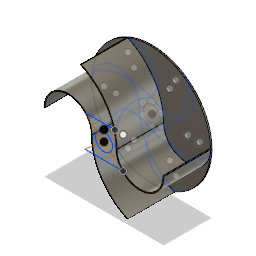
_Urinsky Turbine.044683ae-95bf-4561-8fff-8623c57a335d (Autodesk Fusion 360 design; units mm, degrees)
Autodesk Fusion 360 part; units mm, degrees
sketch "Sketch1" plane through (0, 0, 0) normal (0, 0, 1) x (1, 0, 0)
  circle A0 centre (0, 0) radius 125
  arc A1 (25, -0.0002) -> (-50.0002, 114.5643) centre (-100, -0.0002) ccw
  arc A2 (25, -0.0002) -> (125, -0.0004) centre (75, -0.0002) ccw
  arc A3 (-25, 0.0002) -> (50.0002, -114.5643) centre (100, 0.0002) ccw
  arc A4 (-25, 0.0002) -> (-125, 0.0004) centre (-75, 0.0002) ccw
  arc A5 (27, -0.0002) -> (-47.4802, 115.6314) centre (-100, -0.0002) ccw
  arc A6 (27, -0.0002) -> (123, -0.0004) centre (75, -0.0002) ccw
  arc A7 (-27, 0.0002) -> (47.4802, -115.6314) centre (100, 0.0002) ccw
  arc A8 (-27, 0.0002) -> (-123, 0.0004) centre (-75, 0.0002) ccw
  line L0 (50.0002, -114.5643) -> (47.4802, -115.6314)
  line L1 (-123, 0.0004) -> (-124.9746, -2.5191)
  line L2 (123, -0.0004) -> (124.9746, 2.5191)
  circle A9 centre (0, 0) radius 17.65
  circle A10 centre (0, 22) radius 1.5
  circle A11 centre (-19.0526, 11) radius 1.5
  circle A12 centre (-19.0526, -11) radius 1.5
  circle A13 centre (0, -22) radius 1.5
  circle A14 centre (19.0526, -11) radius 1.5
  circle A15 centre (19.0526, 11) radius 1.5
  line L3 (125, -0.0004) -> (124.9746, 2.5191)
  line L4 (-124.9746, -2.5191) -> (-125, 0.0004)
  line L5 (-50.0002, 114.5643) -> (-47.4802, 115.6314)
  arc A16 (-13.4998, 23.3828) -> (-61.4996, 106.5213) centre (-37.4998, 64.952) ccw
  line L6 (-62.4996, 108.2534) -> (-64.6689, 106.9717)
  line L7 (-61.4996, 106.5213) -> (-64.6689, 106.9717)
  line L8 (74.2155, 100.5836) -> (76.3997, 98.9348)
  line L9 (-74.2155, -100.5836) -> (-76.3997, -98.9348)
  arc A17 (12.4998, -21.6507) -> (62.4996, -108.2534) centre (37.4998, -64.952) ccw
  line L10 (64.6689, -106.9717) -> (62.4996, -108.2534)
  line L11 (61.4996, -106.5213) -> (64.6689, -106.9717)
  arc A18 (13.4998, -23.3828) -> (61.4996, -106.5213) centre (37.4998, -64.952) ccw
  arc A19 (-13.4998, 23.3828) -> (-76.3997, -98.9348) centre (50.0002, -86.6025) ccw
  arc A20 (-12.4998, 21.6507) -> (-74.2155, -100.5836) centre (50.0002, -86.6025) ccw
  arc A21 (-12.4998, 21.6507) -> (-62.4996, 108.2534) centre (-37.4998, 64.952) ccw
  arc A22 (12.4998, -21.6507) -> (74.2155, 100.5836) centre (-50.0002, 86.6025) ccw
  arc A23 (13.4998, -23.3828) -> (76.3997, 98.9348) centre (-50.0002, 86.6025) ccw
  arc A24 (-13.5002, -23.3826) -> (-61.5004, -106.5209) centre (-37.5002, -64.9518) ccw
  line L12 (-62.5004, -108.253) -> (-60.3057, -109.4907)
  line L13 (-61.5004, -106.5209) -> (-60.3057, -109.4907)
  line L14 (-124.2157, 13.9807) -> (-123.8799, 16.6967)
  line L15 (124.2157, -13.9807) -> (123.8799, -16.6967)
  arc A25 (12.5002, 21.6505) -> (62.5004, 108.253) centre (37.5002, 64.9518) ccw
  line L16 (60.3057, 109.4907) -> (62.5004, 108.253)
  line L17 (61.5004, 106.5209) -> (60.3057, 109.4907)
  arc A26 (13.5002, 23.3826) -> (61.5004, 106.5209) centre (37.5002, 64.9518) ccw
  arc A27 (-13.5002, -23.3826) -> (123.8799, -16.6967) centre (49.9998, 86.6026) ccw
  arc A28 (-12.5002, -21.6505) -> (124.2157, -13.9807) centre (49.9998, 86.6026) ccw
  arc A29 (-12.5002, -21.6505) -> (-62.5004, -108.253) centre (-37.5002, -64.9518) ccw
  arc A30 (12.5002, 21.6505) -> (-124.2157, 13.9807) centre (-49.9998, -86.6026) ccw
  arc A31 (13.5002, 23.3826) -> (-123.8799, 16.6967) centre (-49.9998, -86.6026) ccw
  dimension "d1" = 250
  dimension "d2" = 100
  dimension "d3" = 250
  dimension "d5" = 360
  dimension "d8" = 35.3
  dimension "d10" = 3
  dimension "d12" = 360
  dimension "d18" = 360
  measures "d1" diameter of A0
  measures "d2" diameter of A2
  measures "d3" diameter of A1
  measures "d8" diameter of A9
  measures "d10" diameter of A10
extrude "Extrude2" add sketch "Sketch1" along normal blind 100 contours A2 A6 L2 L3 A28 | A2 A6 A27 A28 | A2 A6 A27 | A2 A6 A27 A28 | A2 A6 A23 A28 | A2 A6 A22 A23 | A3 A7 L0 A17 | A3 A7 A17 A18 | A3 A7 A18 | A3 A7 A17 A18 | A1 A2 A5 A6 A22 A25 | A1 A5 L5 A21 | A1 A5 A25 A26 | A3 A7 A17 A24 | A1 A5 A16 A21 | A1 A5 A21 A26 | A3 A7 A24 A29 | A1 A5 A16 | A1 A5 A16 A21 | A3 A4 A7 A8 A20 A29 | A4 A8 A19 A20 | A4 A8 A30 A31 | A4 A8 A31 | A4 A8 A30 A31 | A4 A8 A19 A30 | A4 A8 L1 L4 A30 makes body 1 at (-113.1168, 32.3593, 66.6667) makes body 2 at (111.5588, -34.1097, 66.6667)
extrude "Extrude1" add sketch "Sketch1" along normal blind 3 separate body contours A0 A2 A28 | A0 A6 L2 A23 A25 A28 | A0 L15 | A2 L15 A27 A28 | A0 L8 | L8 A22 A23 A25 | A0 A2 A3 L11 A18 A27 | A6 A27 A28 | A0 A22 A25 | A23 A25 A26 | A22 A23 A25 A26 | A0 L10 | A3 A17 L10 L11 A18 | A2 A18 A27 A28 | A6 A27 | A0 L16 | A22 A25 L16 L17 A26 | A23 A26 | A22 A23 A26 | A22 A23 A25 A26 | A6 A22 A23 A25 | A0 A3 A17 | A2 A18 A23 A28 | A17 A18 A27 A28 | A3 A17 A18 A27 | A0 A5 A21 A22 L17 A26 | A5 A22 A25 A26 | A5 A6 A22 A25 | A2 A17 A18 A22 A23 A28 | A3 A17 A24 A27 A28 A29 | A3 A17 A24 A27 | A0 A7 A17 A20 A24 L13 | A7 A17 A18 | A7 A18 | A1 A2 A3 A4 A17 A20 A21 A22 A25 A28 A29 A30 | A0 A1 A21 | A5 A16 A21 | A1 A21 A25 A26 A30 A31 | A0 L12 | A20 A24 L12 L13 A29 | A0 L6 | A1 A16 L6 L7 A21 | A5 A16 | A1 A21 A26 A31 | A0 A20 A29 | A7 A20 A24 A29 | A0 A1 A4 A16 L7 A31 | A1 A16 A21 A31 | A16 A21 A30 A31 | A4 A16 A19 A20 A21 A30 | A0 L9 | L9 A19 A20 A29 | A19 A20 A24 A29 | A19 A20 A24 | A7 A8 A20 A29 | A19 A20 A24 A29 | A0 L14 | A4 L14 A30 A31 | A4 A16 A30 A31 | A4 A16 A19 A30 | A0 A8 L1 A19 A29 A30 | A19 A24 A29 | A19 A24 | A8 A19 A20 A29 | A0 A4 A30 | A8 A30 A31 | A8 A31 makes body 3 at (83, -13.8567, 0) makes body 4 at (52.2444, -86.2769, 0) makes body 5 at (-63.0924, 13.2677, 0)
combine "Combine1" operation add target body 1 tool bodies 2 3 4 5
sketch "Sketch2" plane through (0, 0, 100) normal (0, 0, 1) x (1, 0, 0)
  arc A0 (25, -0.0002) -> (125, -0.0004) centre (75, -0.0002) ccw
  line L0 (125, -0.0004) -> (124.9746, 2.5191)
  line L1 (124.9746, 2.5191) -> (123, -0.0004)
  arc A1 (27, -0.0002) -> (123, -0.0004) centre (75, -0.0002) ccw
  arc A2 (27, -0.0002) -> (-47.4802, 115.6314) centre (-100, -0.0002) ccw
  line L2 (-47.4802, 115.6314) -> (-50.0002, 114.5643)
  arc A3 (25, -0.0002) -> (-50.0002, 114.5643) centre (-100, -0.0002) ccw
  circle A4 centre (0, 0) radius 17.65
  circle A5 centre (0, 22) radius 1.5
  line L3 (-40, 33) -> (22.6376, 33)
  line L4 (40, -32.8484) -> (40, -33)
  line L5 (40, -33) -> (-40, -33)
  line L6 (-40, 33) -> (40, -33) construction
  line L7 (40, 33) -> (-40, -33) construction
  dimension "d19" = 35.3
  dimension "d20" = 3
  measures "d19" diameter of A4
  measures "d20" diameter of A5
equation "d2 = ( 250 * 0.4 ) * 1 mm"
